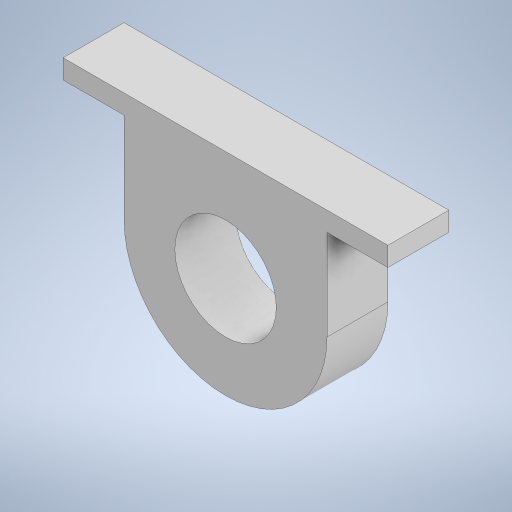
# Autodesk Inventor part: wheel holder
Saved by Autodesk Inventor 2024 (Build 280153000, 153)
## iProperties
Created: 2024-04-10
Part Number: wheel holder
Material: Generic
Document SubType Name: Modeling
Designer: teeta
Density: 1 g/cm^3
Appearance: Default
Author: teeta
Autodesk Inventor part; units mm, degrees
ref_plane "YZ Plane" through (0, 0, 0) normal (1, 0, 0) x (0, 1, 0)
ref_plane "XZ Plane" through (0, 0, 0) normal (0, 1, 0) x (-1, 0, 0)
ref_plane "XY Plane" through (0, 0, 0) normal (0, 0, 1) x (1, 0, 0)
sketch "Sketch1" plane through (0, 0, 0) normal (0, 0, 1) x (1, 0, 0)
  arc A0 (-50, 50) -> (0, 0) centre (0, 50) ccw
  line L0 (0, 0) -> (0, 52.848) construction
  line L1 (0, 0) -> (-10.7104, 0) construction
  arc A1 (0, 0) -> (50, 50) centre (0, 50) ccw
  circle A2 centre (0, 50) radius 25
  arc A3 (0, 25) -> (25, 50) centre (0, 50) ccw
  line L2 (-50, 50) -> (-50, 85)
  line L3 (50, 50) -> (50, 85)
  line L4 (50, 85) -> (-50, 85)
  dimension "d0" = 50
  dimension "d1" = 25
  dimension "d15" = 85
  constraints: 10 end point, 7 point on circle, 4 centre point, 3 vertical, 2 horizontal, 2 tangent, 1 symmetric about line, 1 other
  measures "d0" radius of A0
  measures "d1" radial gap between concentric circles of A0 A2
  measures "d15" distance from line of L0.start L4
extrude "Extrusion1" add sketch "Sketch1" along normal mid plane 30
sketch "Sketch5" plane through (-50, 85, 15) normal (0, 1, 0) x (1, 0, 0)
  line L0 (100, 30) -> (100, 0) projected
  line L1 (100, 30) -> (130, 30)
  line L2 (130, 30) -> (130, 0)
  line L3 (130, 0) -> (100, 0)
  line L4 (100, 0) -> (100, 30)
  line L5 (0, 30) -> (0, 0) projected
  line L6 (0, 30) -> (-30, 30)
  line L7 (-30, 30) -> (-30, 0)
  line L8 (-30, 0) -> (0, 0)
  line L9 (0, 0) -> (0, 30)
  point P0 (50, 15)
  dimension "d16" = 30
  dimension "d17" = 30
  dimension "d18" = 30
  dimension "d19" = 30
  constraints: 16 end point, 4 parallel, 2 horizontal, 2 perpendicular
  measures "d16" distance of L1.end L2.end
  measures "d17" distance of L0.start L1.end
  measures "d18" distance of L7.end L8.end
  measures "d19" distance of L6.end L7.end
extrude "Extrusion4" add sketch "Sketch5" against normal blind 6
move faces "Move1" translate (0, 25.99, 0) faces at (-26.6667, 85, -5)
move faces "Move2" translate (0, 22.5, 0) faces at (-70, 79, -5) (60, 79, -5)
move faces "Move3" translate (0, -6.83, 0) faces at (1.0045, 92.6059, 15) (1.0045, 92.6059, -15) (26.6667, 110.99, 5) (-80, 107.8267, -5) (80, 107.8267, 5) (60, 101.5, -5) (-70, 101.5, -5)
body "Solid1"
